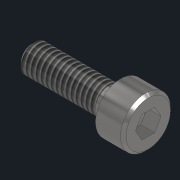
# Autodesk Inventor part: CB2_5-8
Saved by Autodesk Inventor 2022 (Build 260153000, 153)
## iProperties
Category: PARTsolutions
Company: MISUMI
Part Number: CB2_5-8
Material: 鋼、炭素鋼
Catalog Web Link: www.cadenas.de
Description: 在庫有
Vendor: MISUMI
Document SubType Name: Modeling
Designer: partserver
Manufacturer: MISUMI
Mass: 0.578682 g
Surface Area: 1.35234 cm^2
Volume: 0.0737174 cm^3
Density: 7.85 g/cm^3
Appearance: 半つや出し
PSOL_IDENT_0: {$CADENAS_DATA\23d-libs\misumi\metric\27_screws_nuts\cb_fa.prj},152 {VTYP=3D},{NB=CB2.5-8},{LINA=CB2
PSOL_IDENT_1: .5-8},{NN=CB},{DATE=09.09.2019 15:27:56},{GEOMDATE=17.02.2014 00:00:00},{VERSION=},{LINEID=30},{WBVA
PSOL_IDENT_2: R=L},{WBNUMERIC=L}  {NB=CB2.5-8},{LINA=CB2.5-8},{KT=DUMMY},{PN=CB2.5-8},{MAT=4137 Steel},{HARD=38~43
PSOL_IDENT_3: HRC},{ST=Black Oxide},{M=2.5},{L=8},{LL=Full Thread},{L1=60},{TYPE=CB},{M1=2.500},{L0=4,5,6,8,10,12,
PSOL_IDENT_4: 15},{NDM=2.5},{KDM=1.947099},{MP=2.5x0.45},{P=0.45},{A=4.5},{E=2.5},{B=2.0},{V=0.25}
NB: CB2.5-8
NN: CB
NT: Hexagon Socket Head Cap Screws
NBSYN: $PN.
LINA: CB2.5-8
CATALOG: Misumi
PN: CB2.5-8
MAT: 4137 Steel
HARD: 38~43HRC
ST: Black Oxide
M: 2.5
L: 8
LL: Full Thread
MP: 2.5x0.45
A: 4.5
E: 2.5
B: 2
SUPPLIER: MISUMI
ARTICLENO: CB2.5-8
BOMINFO: CB2.5-8
CREATOR: CADENAS GmbH
Title: CB2.5-8
Author: Cadenas PARTsolutions
Comments: Hexagon Socket Head Cap Screws
Autodesk Inventor part; units mm, degrees
sketch "Sketch_1" plane through (0, 0, 0) normal (0, 0, 1) x (1, 0, 0)
  line L0 (8, 0) -> (-2.5, 0)
  line L1 (-2.5, 0) -> (-2.5, 2)
  line L2 (-2.5, 2) -> (-2.25, 2.25)
  line L3 (-2.25, 2.25) -> (0, 2.25)
  line L4 (0, 2.25) -> (0, 1.25)
  line L5 (0, 1.25) -> (7.724, 1.25)
  line L6 (7.724, 1.25) -> (8, 0.974)
  line L7 (8, 0.974) -> (8, 0)
  line L8 (8, 0) -> (-2.5, 0)
  constraints: 18 end point
revolve "Revolution1" add sketch "Sketch_1" angle 360 about axis through (8, 0, 0) along (1, 0, 0)
thread "Thread1" size "M2.5x0.45" class "6g" standard "ISO Metric profile" length 6.724
sketch "Sketch2" plane through (-2.5, 0, 0) normal (-1, 0, 0) x (0, 0, 1)
  point P0 (0, 0)
hole "Hole1" at (-2.5, 0, 0) direction (1, 0, 0) diameter 2 depth 1.25 tip angle 150
sketch "Sketch_3" plane through (-2.5, 0, 0) normal (1, 0, 0) x (0, 0, -1)
  line L0 (-1, -0.5774) -> (0, -1.1547)
  line L1 (0, -1.1547) -> (1, -0.5774)
  line L2 (1, -0.5774) -> (1, 0.5774)
  line L3 (1, 0.5774) -> (0, 1.1547)
  line L4 (0, 1.1547) -> (-1, 0.5774)
  line L5 (-1, 0.5774) -> (-1, -0.5774)
  constraints: 12 end point
extrude "Extrusion1" cut sketch "Sketch_3" along normal blind 1.25
ref_plane "bolt_to_nut_XY" through (8, 0, 0) normal (1, 0, 0) x (0, 0, -1)
ref_plane "bolt_to_nut_YZ" through (8, 0, 0) normal (0, 0, -1) x (0, 1, 0)
ref_plane "bolt_to_nut_ZX" through (8, 0, 0) normal (0, 1, 0) x (1, 0, 0)
ref_plane "screw1_XY" through (0, 0, 0) normal (1, 0, 0) x (0, 0, -1)
ref_plane "screw1_YZ" through (0, 0, 0) normal (0, 0, -1) x (0, 1, 0)
ref_plane "screw1_ZX" through (0, 0, 0) normal (0, 1, 0) x (1, 0, 0)
body "Solid1"
